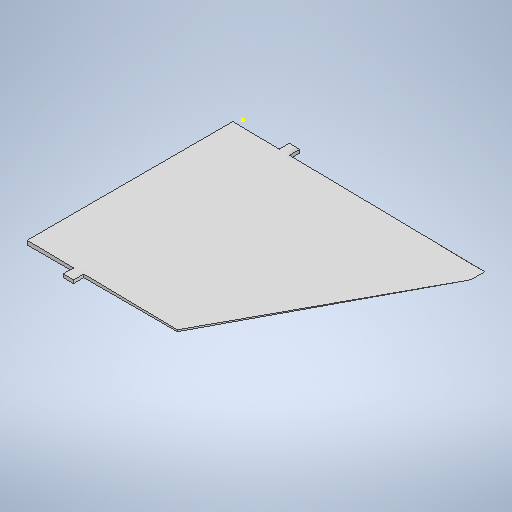
# Autodesk Inventor part: 坂
Saved by Autodesk Inventor 2026.2 (Build 302298010, 298A)
## iProperties
Created: 2026-05-25
Part Number: 坂
Material: 一般
Document SubType Name: Modeling
Designer: Yagis
Density: 1 g/cm^3
Appearance: 既定
Author: Yagis
Autodesk Inventor part; units mm, degrees
ref_plane "YZ Plane" through (0, 0, 0) normal (1, 0, 0) x (0, 1, 0)
ref_plane "XZ Plane" through (0, 0, 0) normal (0, 1, 0) x (-1, 0, 0)
ref_plane "XY Plane" through (0, 0, 0) normal (0, 0, 1) x (1, 0, 0)
sketch "スケッチ1" plane through (0, 0, 0) normal (0, 1, 0) x (-1, 0, 0)
  point P0 (0, 0)
sketch "スケッチ2" plane through (0, 0, 0) normal (0, 0, 1) x (1, 0, 0)
  line L0 (0, 0) -> (0, 4)
  line L1 (0, 4) -> (245, 0)
  line L2 (0, 0) -> (245, 0)
  dimension "d0" = 4
  dimension "d1" = 245
  constraints: 6 end point, 1 horizontal, 1 vertical
  measures "d0" distance of L0.start L0.end
  measures "d1" distance of L0.start L1.end
extrude "押し出し1" add sketch "スケッチ2" along normal blind 220
sketch "スケッチ4" plane through (0, 0, 220) normal (0, 0, 1) x (1, 0, 0)
  line L0 (0, 4) -> (0, 0) projected
  line L1 (55, 0) -> (245, 0)
  line L2 (245, 0) -> (245, 4)
  line L3 (245, 4) -> (55, 4)
  line L4 (55, 4) -> (55, 0)
  line L5 (0, 4) -> (45, 4)
  line L6 (45, 4) -> (45, 0)
  line L7 (45, 0) -> (0, 0)
  line L8 (0, 0) -> (0, 4)
  dimension "d8" = 4
  dimension "d9" = 190
  dimension "d10" = 55
  dimension "d23" = 45
  constraints: 16 end point, 4 parallel, 2 horizontal, 2 perpendicular
  measures "d8" distance between parallel lines of L1 L3
  measures "d9" distance between parallel lines of L2 L4
  measures "d10" distance between parallel lines of L0 L4
  measures "d23" distance of L6.end L7.end
extrude "押し出し2" cut sketch "スケッチ4" against normal blind 10
sketch "スケッチ5" plane through (0, 0, 0) normal (0, 0, -1) x (-1, 0, 0)
  line L0 (-55, 0) -> (-245, 0)
  line L1 (-245, 0) -> (-245, 4)
  line L2 (-245, 4) -> (-55, 4)
  line L3 (-55, 4) -> (-55, 0)
  line L4 (0, 4) -> (0, 0) projected
  line L5 (0, 4) -> (-45, 4)
  line L6 (-45, 4) -> (-45, 0)
  line L7 (-45, 0) -> (0, 0)
  line L8 (0, 0) -> (0, 4)
  dimension "d13" = 4
  dimension "d14" = 55
  dimension "d15" = 190
  dimension "d22" = 45
  constraints: 16 end point, 4 parallel, 2 horizontal, 2 perpendicular
  measures "d13" distance between parallel lines of L2 L0
  measures "d14" distance between parallel lines of L4 L3
  measures "d15" distance of L0.start L0.end
  measures "d22" distance between parallel lines of L6 L4
extrude "押し出し3" cut sketch "スケッチ5" against normal blind 10
sketch "スケッチ6" plane through (0, 0, 0) normal (0, -1, 0) x (1, 0, 0)
  line L0 (0, 0) -> (0, 220) projected
  line L1 (55, 10) -> (245, 10) projected
  line L2 (245, 23.5) -> (146, 210)
  line L3 (245, 210) -> (245, 23.5)
  line L4 (146, 210) -> (245, 23.5)
  line L5 (146, 210) -> (245, 210)
  line L6 (245, 210) -> (55, 210) projected
  dimension "d18" = 146
  dimension "d19" = 13.5
  constraints: 8 end point, 1 collinear, 1 horizontal, 1 vertical
  measures "d18" distance from line of L0 L2.end
  measures "d19" distance from line of L1 L2.start
extrude "押し出し4" cut sketch "スケッチ6" against normal blind 10
